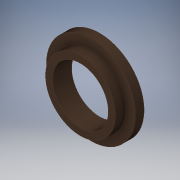
# Autodesk Inventor part: Seat
Saved by Autodesk Inventor 2018 (Build 220112000, 112)
## iProperties
Created: 2017-09-07
Part Number: Seat
Material: Bronze, Soft Tin
Document SubType Name: Modeling
Designer: kurtis
Density: 8.874 g/cm^3
Appearance: Bronze - Satin
Author: kurtis
Autodesk Inventor part; units mm, degrees
ref_plane "YZ Plane" through (0, 0, 0) normal (1, 0, 0) x (0, 1, 0)
ref_plane "XZ Plane" through (0, 0, 0) normal (0, 1, 0) x (-1, 0, 0)
ref_plane "XY Plane" through (0, 0, 0) normal (0, 0, 1) x (1, 0, 0)
sketch "Sketch1" plane through (0, 0, 0) normal (0, 0, 1) x (1, 0, 0)
  line L0 (0, 0) -> (16, 0) construction
  line L1 (16, 0) -> (16, 11)
  line L2 (16, 11) -> (25.5, 11)
  line L3 (25.5, 11) -> (25.5, 6)
  line L4 (16, 0) -> (20, 0)
  line L5 (20, 0) -> (20, 6)
  line L6 (20, 6) -> (25.5, 6)
  line L7 (0, 0) -> (0, 17.5588) construction
  dimension "d0" = 16
  dimension "d1" = 11
  dimension "d2" = 9.5
  dimension "d3" = 5
  dimension "d4" = 4
  constraints: 16 end point, 4 perpendicular, 2 horizontal, 2 vertical
  measures "d0" distance of L0.start L0.end
  measures "d1" distance of L0.end L1.end
  measures "d2" distance of L1.end L2.end
  measures "d3" distance of L2.end L3.end
  measures "d4" distance of L0.end L4.end
revolve "Revolution1" add sketch "Sketch1" angle 360 about axis through (0, 0, 0) along (0, 1, 0)
body "Solid1"
